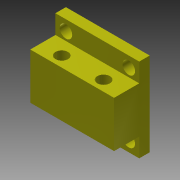
# Autodesk Inventor part: Conector
Saved by Autodesk Inventor 2015 (Build 190159000, 159)
## iProperties
Created: 2016-01-15
Part Number: Conector
Material: Generic
Document SubType Name: Modeling
Designer: david
Density: 1 g/cm^3
Appearance: Yellow
Author: david
Autodesk Inventor part; units mm, degrees
ref_plane "YZ Plane" through (0, 0, 0) normal (1, 0, 0) x (0, 1, 0)
ref_plane "XZ Plane" through (0, 0, 0) normal (0, 1, 0) x (-1, 0, 0)
ref_plane "XY Plane" through (0, 0, 0) normal (0, 0, 1) x (1, 0, 0)
sketch "Sketch1" plane through (0, 0, 0) normal (0, 1, 0) x (-1, 0, 0)
  line L0 (-20, -11) -> (20, -11)
  line L1 (20, -11) -> (20, 11)
  line L2 (20, 11) -> (-20, 11)
  line L3 (-20, 11) -> (-20, -11)
  line L4 (-20, -11) -> (20, 11) construction
  line L5 (20, -11) -> (-20, 11) construction
  point P0 (0, 0)
  dimension "d0" = 22
  dimension "d1" = 40
  constraints: 12 end point, 2 midpoint, 2 parallel, 1 horizontal, 1 perpendicular
  measures "d0" distance of L0.end L1.end
  measures "d1" distance of L0.start L0.end
extrude "Extrusion1" add sketch "Sketch1" along normal blind 12
sketch "Sketch2" plane through (0, 12, 0) normal (0, 1, 0) x (1, 0, 0)
  line L0 (20, -20) -> (-20, -20)
  line L1 (-20, -20) -> (-20, 20)
  line L2 (-20, 20) -> (20, 20)
  line L3 (20, 20) -> (20, -20)
  line L4 (20, -20) -> (-20, 20) construction
  line L5 (-20, -20) -> (20, 20) construction
  point P0 (0, 0)
  dimension "d4" = 40
  dimension "d5" = 40
  constraints: 12 end point, 2 midpoint, 2 parallel, 1 horizontal, 1 perpendicular
  measures "d4" distance of L0.end L1.end
  measures "d5" distance of L1.end L2.end
extrude "Extrusion2" add sketch "Sketch2" along normal blind 5
sketch "Sketch3" plane through (0, 17, 0) normal (0, 1, 0) x (1, 0, 0)
  circle A0 centre (-15, -15) radius 3
  line L0 (-20, -20) -> (20, -20) projected
  line L1 (-20, 20) -> (-20, -20) projected
  circle A1 centre (15, -15) radius 3
  circle A2 centre (15, 15) radius 3
  circle A3 centre (-15, 15) radius 3
  line L2 (-20, 20) -> (20, 20) projected
  line L3 (20, -20) -> (20, 20) projected
  point P0 (0, 0)
  dimension "d8" = 6
  dimension "d9" = 5
  dimension "d10" = 5
  dimension "d11" = 6
  dimension "d12" = 6
  dimension "d13" = 6
  dimension "d14" = 5
  dimension "d15" = 5
  dimension "d16" = 5
  dimension "d17" = 5
  dimension "d18" = 5
  dimension "d19" = 5
  constraints: 4 centre point
  measures "d8" diameter of A0
  measures "d9" distance from line of L0 A0.centre
  measures "d10" distance from line of L1 A0.centre
  measures "d11" diameter of A1
  measures "d12" diameter of A2
  measures "d13" diameter of A3
  measures "d14" distance from line of L1 A3.centre
  measures "d15" distance from line of L2 A3.centre
  measures "d16" distance from line of L2 A2.centre
  measures "d17" distance from line of L3 A2.centre
  measures "d18" distance from line of L3 A1.centre
  measures "d19" distance from line of L0 A1.centre
extrude "Extrusion3" cut sketch "Sketch3" against normal blind 100 keep common part
sketch "Sketch4" plane through (-20, 0, 11) normal (0, 0, 1) x (1, 0, 0)
  circle A0 centre (10, 5) radius 3
  circle A1 centre (30, 5) radius 3
  line L0 (0, 0) -> (0, 12) projected
  line L1 (40, 0) -> (40, 12) projected
  line L2 (40, 0) -> (0, 0) projected
  point P0 (20, 0)
  dimension "d22" = 6
  dimension "d23" = 6
  dimension "d24" = 10
  dimension "d25" = 10
  dimension "d26" = 5
  dimension "d27" = 5
  constraints: 2 centre point
  measures "d22" diameter of A0
  measures "d23" diameter of A1
  measures "d24" distance from line of L0 A0.centre
  measures "d25" distance from line of L1 A1.centre
  measures "d26" distance from line of L2 A1.centre
  measures "d27" distance from line of L2 A0.centre
extrude "Extrusion4" cut sketch "Sketch4" against normal blind 100
body "Solid1"
